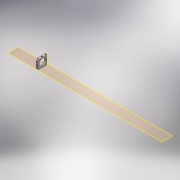
# Autodesk Inventor part: x-box-rib-10
Saved by Autodesk Inventor 2016 (Build 200138000, 138)
## iProperties
Created: 2015-05-14
Part Number: x-box-rib-10
Material: Generic
Document SubType Name: Modeling
Designer: as
Density: 1 g/cm^3
Appearance: Default
Mass: 13.9344 g
Surface Area: 71.9457 cm^2
Volume: 13.9344 cm^3
Author: as
Autodesk Inventor part; units mm, degrees
ref_plane "YZ Plane" through (0, 0, 0) normal (1, 0, 0) x (0, 1, 0)
ref_plane "Work Plane1" through (275, -2.5, 0) normal (0, 0, 1) x (1, 0, 0)
sketch "Sketch1" plane through (275, -2.5, 0) normal (0, 0, 1) x (1, 0, 0)
  line L0 (-280, -25) -> (-280, 30)
  line L1 (-280, 30) -> (-270, 30)
  line L2 (-270, 30) -> (-270, -25)
  line L3 (-270, -25) -> (-280, -25)
  line L4 (-280, -25) -> (-270, 30) construction
  line L5 (-280, 30) -> (-270, -25) construction
  point P0 (-275, 2.5)
  dimension "d0" = 55
  dimension "d1" = 10
  constraints: 12 end point, 2 midpoint, 2 parallel, 1 perpendicular, 1 vertical
  measures "d0" distance of L0.start L0.end
  measures "d1" distance of L0.end L1.end
ref_plane "Work Plane2" through (-400, -24, 0) normal (0, 0, 1) x (1, 0, 0)
ref_plane "Work Plane3" through (-400, -24, 50) normal (0, 0, -1) x (0, 1, 0)
extrude "Extrusion1" add sketch "Sketch1" along normal up to surface (50 mm away) from surface at 0
sketch "Sketch2" plane through (5, -27.5, 50) normal (1, 0, 0) x (0, 0, -1)
  circle A0 centre (25, 27.5) radius 20
  line L0 (50, 55) -> (50, 0) projected
  line L1 (0, 0) -> (50, 0) projected
  point P0 (50, 27.5)
  dimension "d4" = 40
  dimension "d5" = 25
  dimension "d6" = 27.5
  constraints: 1 centre point
  measures "d4" diameter of A0
  measures "d5" distance from line of L0 A0.centre
  measures "d6" distance from line of L1 A0.centre
extrude "Extrusion2" cut sketch "Sketch2" against normal through all
sketch "Sketch3" plane through (-5, 27.5, 50) normal (0, 0, 1) x (1, 0, 0)
  line L0 (10, 0) -> (0, 0) projected
  line L1 (0, -55) -> (10, -55) projected
  point P0 (5, -27.5)
  point P1 (5, -27.5)
  point P2 (5, -5)
  point P3 (5, -50)
  dimension "d12" = 5
  dimension "d13" = 5
  dimension "d14" = 22.5
  dimension "d15" = 22.5
  constraints: 1 coincident
  measures "d12" distance from line of L0 point (5, -5)
  measures "d13" distance from line of L1 point (5, -50)
  measures "d14" distance of point (5, -5) point (5, -27.5)
  measures "d15" distance of point (5, -50) point (5, -27.5)
sketch "Sketch4" plane through (-5, 27.5, 50) normal (0, 1, 0) x (1, 0, 0)
  line L0 (10, 45) -> (0, 45) projected
  line L1 (0, 50) -> (10, 50) projected
  line L2 (10, 0) -> (0, 0) projected
  line L3 (10, 0) -> (10, 50) projected
  point P0 (5, 50)
  point P1 (5, 25)
  dimension "d17" = 25
  dimension "d21" = 5
  measures "d17" distance from line of L1 point (5, 25)
  measures "d21" distance from line of point (5, 25) L3
sketch "Sketch5" plane through (5, 27.5, 0) normal (0, 0, -1) x (-1, 0, 0)
  line L0 (10, 0) -> (0, 0) projected
  line L1 (0, -55) -> (10, -55) projected
  point P0 (5, -27.5)
  point P1 (5, -27.5)
  point P2 (5, -5)
  point P3 (5, -50)
  dimension "d22" = 22.5
  dimension "d23" = 27.5
  dimension "d24" = 5
  dimension "d25" = 22.5
  dimension "d26" = 5
  constraints: 1 coincident
  measures "d22" distance of point (5, -27.5) point (5, -50)
  measures "d23" distance from line of L0 point (5, -27.5)
  measures "d24" distance from line of L0 point (5, -5)
  measures "d25" distance of point (5, -27.5) point (5, -5)
  measures "d26" distance from line of L1 point (5, -50)
sketch "Sketch6" plane through (-5, -27.5, 50) normal (0, -1, 0) x (1, 0, 0)
  line L0 (0, 0) -> (10, 0) projected
  point P0 (5, -50)
  point P1 (5, -25)
  dimension "d27" = 25
  dimension "d28" = 25
  measures "d27" distance of point (5, -50) point (5, -25)
  measures "d28" distance from line of L0 point (5, -25)
sketch "Sketch11" plane through (5, 27.5, 0) normal (0, 0, -1) x (-1, 0, 0)
  point P0 (3, -50)
  point P1 (303, -27.5)
  point P2 (303, -50)
  point P3 (303, -5)
  point P4 (603, -5)
  point P5 (603, -27.5)
  point P6 (603, -50)
  point P7 (3, -5)
  point P8 (3, -27.5)
hole "Hole9" at (2, -22.5, 0) at (-298, 0, 0) at (-298, -22.5, 0) at (-298, 22.5, 0) at (-598, 22.5, 0) at (-598, 0, 0) at (-598, -22.5, 0) at (2, 22.5, 0) at (2, 0, 0) direction (0, 0, 1) diameter 4.134 depth 12 tip angle 120 thread size "M5x0.8" class "6H" standard "ISO Metric profile"
sketch "Sketch12" plane through (-5, 27.5, 50) normal (0, 0, 1) x (1, 0, 0)
  point P0 (5, -27.5)
  point P1 (5, -5)
  point P2 (5, -50)
  point P3 (-295, -50)
  point P4 (-295, -27.5)
  point P5 (-295, -5)
  point P6 (-595, -27.5)
  point P7 (-595, -5)
  point P8 (-595, -50)
hole "Hole11" at (0, 0, 50) at (0, 22.5, 50) at (0, -22.5, 50) at (-300, -22.5, 50) at (-300, 0, 50) at (-300, 22.5, 50) at (-600, 0, 50) at (-600, 22.5, 50) at (-600, -22.5, 50) direction (0, 0, -1) diameter 4.134 depth 12 tip angle 120 thread size "M5x0.8" class "6H" standard "ISO Metric profile"
hole "Hole15" at (0, -27.5, 25) direction (0, 1, 0) diameter 4.134 end through all thread size "M5x0.8" class "6H" standard "ISO Metric profile"
sketch "Sketch14" plane through (-5, -27.5, 50) normal (0, -1, 0) x (1, 0, 0)
  point P0 (5, -25)
sketch "Sketch15" plane through (-5, 27.5, 50) normal (0, 1, 0) x (1, 0, 0)
  point P0 (5, 25)
hole "Hole18" at (0, 27.5, 25) direction (0, -1, 0) diameter 4.134 depth 13 tip angle 120 thread size "M5x0.8" class "6H" standard "ISO Metric profile"
equation "\"d6\" = 0.5 * d0"
body "Solid1"
